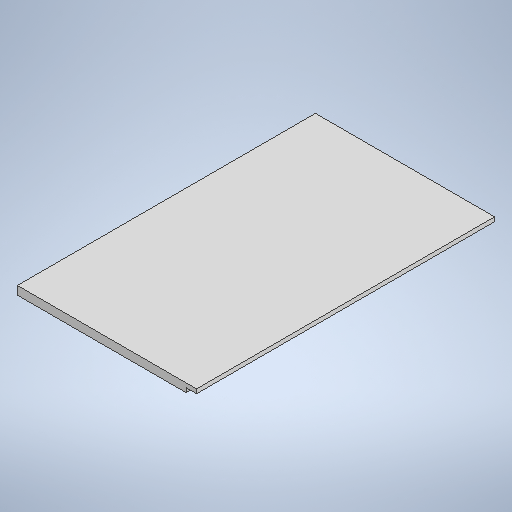
# Autodesk Inventor part: side_wall
Saved by Autodesk Inventor 2026.1 (Build 301233000, 233)
## iProperties
Created: 2026-08-11
Part Number: side_wall
Material: Generic
Document SubType Name: Modeling
Designer: rowan
Density: 1 g/cm^3
Appearance: Default
Author: rowan
Autodesk Inventor part; units mm, degrees
ref_plane "YZ Plane" through (0, 0, 0) normal (1, 0, 0) x (0, 1, 0)
ref_plane "XZ Plane" through (0, 0, 0) normal (0, 1, 0) x (-1, 0, 0)
ref_plane "XY Plane" through (0, 0, 0) normal (0, 0, 1) x (1, 0, 0)
sketch "Sketch1" plane through (0, 0, 0) normal (0, 1, 0) x (-1, 0, 0)
  line L0 (0, 0) -> (80, 0)
  line L1 (80, 0) -> (80, -141.4)
  line L2 (80, -141.4) -> (0, -141.4)
  line L3 (0, -141.4) -> (0, 0)
  dimension "d0" = 80
  dimension "d1" = 141.4
  constraints: 8 end point, 2 parallel, 1 horizontal, 1 perpendicular
  measures "d0" distance of L1.end L2.end
  measures "d1" distance of L2.end L0.start
extrude "Extrusion1" add sketch "Sketch1" along normal blind 4
sketch "Sketch2" plane through (0, 4, 0) normal (0, 1, 0) x (1, 0, 0)
  line L0 (0, 0) -> (0, 141.4) projected
  line L1 (0, 0) -> (5, 0)
  line L2 (5, 0) -> (5, 141.4)
  line L3 (5, 141.4) -> (0, 141.4)
  line L4 (0, 141.4) -> (0, 0)
  dimension "d4" = 5
  constraints: 8 end point, 2 parallel, 1 horizontal, 1 perpendicular
  measures "d4" distance of L0.start L1.end
extrude "Extrusion2" add sketch "Sketch2" against normal blind 2
body "Solid1"
